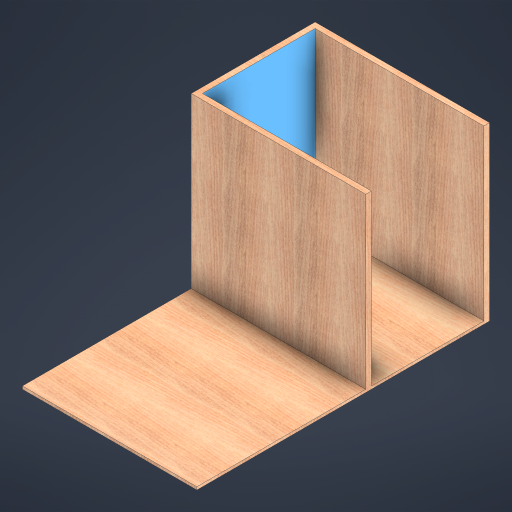
# Autodesk Inventor part: Stage
Saved by Autodesk Inventor 2023 (Build 270158000, 158)
## iProperties
Created: 2023-07-25
Part Number: Stage
Material: Wood (Birch)
Document SubType Name: Modeling
Designer: Abhinav
Density: 0.55 g/cm^3
Appearance: Birch - Natural Polished
Author: Abhinav
Autodesk Inventor part; units mm, degrees
ref_plane "YZ Plane" through (0, 0, 0) normal (1, 0, 0) x (0, 1, 0)
ref_plane "XZ Plane" through (0, 0, 0) normal (0, 1, 0) x (-1, 0, 0)
ref_plane "XY Plane" through (0, 0, 0) normal (0, 0, 1) x (1, 0, 0)
sketch "Sketch1" plane through (0, 0, 0) normal (0, 1, 0) x (-1, 0, 0)
  line L0 (300, 200) -> (-300, 200)
  line L1 (-300, 200) -> (-300, -200)
  line L2 (-300, -200) -> (300, -200)
  line L3 (300, -200) -> (300, 200)
  line L4 (300, 200) -> (-300, -200) construction
  line L5 (-300, 200) -> (300, -200) construction
  line L6 (320, 220) -> (-320, 220)
  line L7 (-320, 220) -> (-320, 200)
  line L8 (-300, -220) -> (320, -220)
  line L9 (320, -220) -> (320, 220)
  line L10 (320, 220) -> (-320, -220) construction
  line L11 (-320, 220) -> (320, -220) construction
  line L12 (-300, -200) -> (-300, -220)
  line L13 (-300, 200) -> (-300, 220)
  point P0 (0, 0)
  dimension "d0" = 600
  dimension "d1" = 400
  dimension "d2" = 640
  dimension "d3" = 440
  constraints: 28 end point, 4 midpoint, 4 parallel, 3 perpendicular, 3 point on line, 2 horizontal
  measures "d0" distance of L2.end L1.end
  measures "d1" distance of L1.end L0.end
  measures "d2" distance of L8.end L10.end
  measures "d3" distance of L10.end L6.end
extrude "Extrusion1" add sketch "Sketch1" against normal blind 600 contours L0 L13 L6 L9 L8 L12 L2 L3
sketch "Sketch2" plane through (0, -600, 0) normal (0, -1, 0) x (1, 0, 0)
  line L0 (-320, -220) -> (-320, 220) projected
  line L1 (-320, -220) -> (300, -220)
  line L2 (300, -220) -> (300, 820)
  line L3 (300, 820) -> (-320, 820)
  line L4 (-320, 820) -> (-320, -220)
  point P0 (300, 220)
  point P1 (-320, 220)
  dimension "d14" = 1040
  dimension "d15" = 620
  constraints: 8 end point, 2 parallel, 1 horizontal, 1 perpendicular
  measures "d14" distance of L2.end L1.end
  measures "d15" distance of L2.end L3.end
extrude "Extrusion2" add sketch "Sketch2" along normal blind 10
body "Solid1"
